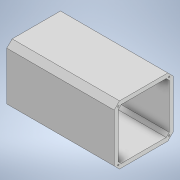
# Autodesk Inventor part: shell
Saved by Autodesk Inventor 2020.3 (Build 243373000, 373)
## iProperties
Created: 2020-08-10
Part Number: shell
Material: Generic
Document SubType Name: Modeling
Designer: joesp
Density: 1 g/cm^3
Appearance: Default
Author: joesp
Autodesk Inventor part; units mm, degrees
ref_plane "YZ Plane" through (0, 0, 0) normal (1, 0, 0) x (0, 1, 0)
ref_plane "XZ Plane" through (0, 0, 0) normal (0, 1, 0) x (-1, 0, 0)
ref_plane "XY Plane" through (0, 0, 0) normal (0, 0, 1) x (1, 0, 0)
sketch "Sketch1" plane through (0, 0, 0) normal (1, 0, 0) x (0, 1, 0)
  line L0 (100, 110) -> (110, 100)
  line L1 (110, 100) -> (110, 10)
  line L2 (110, 10) -> (100, 0)
  line L3 (100, 0) -> (10, 0)
  line L4 (10, 0) -> (0, 10)
  line L5 (0, 10) -> (0, 100)
  line L6 (0, 100) -> (10, 110)
  line L7 (10, 110) -> (100, 110)
  line L8 (102.5, 96.8934) -> (102.5, 13.1066)
  line L9 (96.8934, 7.5) -> (13.1066, 7.5)
  line L10 (13.1066, 7.5) -> (7.5, 13.1066)
  line L11 (7.5, 13.1066) -> (7.5, 96.8934)
  line L12 (7.5, 96.8934) -> (13.1066, 102.5)
  line L13 (13.1066, 102.5) -> (96.8934, 102.5)
  circle A0 centre (102.3483, 7.6517) radius 1.5
  circle A1 centre (102.3483, 102.3483) radius 1.5
  circle A2 centre (7.6517, 102.3483) radius 1.5
  circle A3 centre (7.6517, 7.6517) radius 1.5
  line L14 (96.8934, 7.5) -> (102.5, 13.1066)
  line L15 (102.5, 96.8934) -> (96.8934, 102.5)
  point P0 (0, 0)
  dimension "d0" = 110
  dimension "d1" = 110
  dimension "d2" = 45
  dimension "d3" = 10
  dimension "d4" = 7.5
  dimension "d5" = 7.5
  dimension "d6" = 7.5
  dimension "d7" = 7.5
  dimension "d8" = 45
  dimension "d11" = 3
  dimension "d13" = 3.75
  dimension "d14" = 7.5
  dimension "d15" = 3.75
  dimension "d18" = 8.0039
  dimension "d19" = 8.0039
  dimension "d20" = 7.5
  dimension "d21" = 3.75
  dimension "d22" = 3.75
  dimension "d23" = 8.0039
  dimension "d24" = 8.0039
  dimension "d25" = 3.75
  dimension "d26" = 3.75
  dimension "d27" = 8.0039
  dimension "d28" = 8.0039
  dimension "d29" = 3.75
  dimension "d30" = 3.75
  dimension "d31" = 8.0039
  dimension "d32" = 8.0039
  constraints: 32 end point, 8 equal length, 5 parallel, 5 perpendicular, 4 centre point, 3 equal radius, 1 horizontal alignment, 1 vertical, 1 vertical alignment
  measures "d0" distance between parallel lines of L5 L1
  measures "d1" distance between parallel lines of L3 L7
  measures "d2" angle of L5 L4
  measures "d3" distance of point (0, 0) L3.end
  measures "d4" distance between parallel lines of L1 L8
  measures "d5" distance between parallel lines of L7 L13
  measures "d6" distance between parallel lines of L3 L9
  measures "d7" distance between parallel lines of L5 L11
  measures "d8" angle of L11 L10
  measures "d11" diameter of A0
  measures "d13" distance from line of L2 A0.centre
  measures "d14" distance between parallel lines of L2 L14
  measures "d15" distance from line of L14 A0.centre
  measures "d18" distance of L2.end A0.centre
  measures "d19" distance of L1.end A0.centre
  measures "d20" distance between parallel lines of L0 L15
  measures "d21" distance from line of L0 A1.centre
  measures "d22" distance from line of L15 A1.centre
  measures "d23" distance of L0.end A1.centre
  measures "d24" distance of L0.start A1.centre
  measures "d25" distance from line of L10 A3.centre
  measures "d26" distance from line of L4 A3.centre
  measures "d27" distance of L3.end A3.centre
  measures "d28" distance of L4.end A3.centre
  measures "d29" distance from line of L12 A2.centre
  measures "d30" distance from line of L6 A2.centre
  measures "d31" distance of L6.end A2.centre
  measures "d32" distance of L5.end A2.centre
extrude "Extrusion1" add sketch "Sketch1" along normal blind 200
equation "\"d1\" = d0"
equation "\"d5\" = d4"
equation "\"d6\" = d4"
equation "\"d7\" = d4"
equation "\"d14\" = d4"
equation "\"d15\" = d13"
equation "\"d18\" = d19"
equation "\"d20\" = d4"
equation "\"d21\" = d22"
equation "\"d25\" = d26"
equation "\"d29\" = d30"
body "Solid1"
